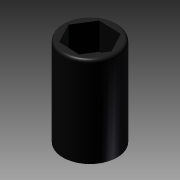
# Autodesk Inventor part: 4
Saved by Autodesk Inventor 2012 (Build 160160000, 160)
## iProperties
Created: 2012-06-13
Part Number: 4
Material: Default
Document SubType Name: Modeling
Designer: Luis
Density: 1 g/cm^3
Author: Luis
Autodesk Inventor part; units mm, degrees
ref_plane "YZ Plane" through (0, 0, 0) normal (1, 0, 0) x (0, 1, 0)
ref_plane "XZ Plane" through (0, 0, 0) normal (0, 1, 0) x (-1, 0, 0)
ref_plane "XY Plane" through (0, 0, 0) normal (0, 0, 1) x (1, 0, 0)
sketch "Sketch1" plane through (0, 0, 0) normal (0, 0, 1) x (1, 0, 0)
  circle A0 centre (0, 0) radius 3
  dimension "d0" = 6
  constraints: 1 centre point, 1 coincident
  measures "d0" diameter of A0
extrude "Extrusion1" add sketch "Sketch1" along normal blind 10
sketch "Sketch2" plane through (0, 0, 10) normal (0, 0, 1) x (1, 0, 0)
  circle A0 centre (0, 0) radius 3 projected
  line L0 (1.3157, 2.1001) -> (2.4766, -0.0894)
  line L1 (2.4766, -0.0894) -> (1.1609, -2.1895)
  line L2 (1.1609, -2.1895) -> (-1.3157, -2.1001)
  line L3 (-1.3157, -2.1001) -> (-2.4766, 0.0894)
  line L4 (-2.4766, 0.0894) -> (-1.1609, 2.1895)
  line L5 (-1.1609, 2.1895) -> (1.3157, 2.1001)
  constraints: 12 end point, 1 coincident, 13 other
extrude "Extrusion2" cut sketch "Sketch2" against normal blind 3 contours L0 L1 L2 L3 L4 L5
fillet "Fillet1" radius 0.3 1 edges at (-3, 0, 10)
body "Solid1"
